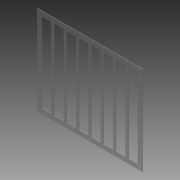
# Autodesk Inventor part: Back Plate Flat
Saved by Autodesk Inventor 2013 (Build 170138000, 138)
## iProperties
Created: 2013-02-02
Part Number: Back Plate Flat
Material: Polycarbonate, Clear
Document SubType Name: Modeling
Designer: Arpan
Mass: 34.1531 g
Surface Area: 558.316 cm^2
Volume: 38.2026 cm^3
Density: 0.894 g/cm^3
Author: Arpan
Autodesk Inventor part; units mm, degrees
ref_plane "YZ Plane" through (0, 0, 0) normal (1, 0, 0) x (0, 1, 0)
ref_plane "XZ Plane" through (0, 0, 0) normal (0, 1, 0) x (-1, 0, 0)
ref_plane "XY Plane" through (0, 0, 0) normal (0, 0, 1) x (1, 0, 0)
sketch "Sketch1" plane through (0, 0, 0) normal (0, 0, 1) x (1, 0, 0)
  line L0 (0, 0) -> (0, 238.1523)
  line L1 (0, 238.1523) -> (282.575, 238.1523)
  line L2 (282.575, 238.1523) -> (282.575, 0)
  line L3 (282.575, 0) -> (0, 0)
  line L4 (12.7, 225.4523) -> (38.1, 225.4523)
  line L5 (12.7, 225.4523) -> (12.7, 12.7)
  line L6 (12.7, 12.7) -> (38.1, 12.7)
  line L7 (38.1, 12.7) -> (38.1, 225.4523)
  line L8 (45.8107, 225.4523) -> (71.2107, 225.4523)
  line L9 (45.8107, 225.4523) -> (45.8107, 12.7)
  line L10 (45.8107, 12.7) -> (71.2107, 12.7)
  line L11 (71.2107, 12.7) -> (71.2107, 225.4523)
  line L12 (78.9214, 225.4523) -> (104.3214, 225.4523)
  line L13 (78.9214, 225.4523) -> (78.9214, 12.7)
  line L14 (78.9214, 12.7) -> (104.3214, 12.7)
  line L15 (104.3214, 12.7) -> (104.3214, 225.4523)
  line L16 (112.0321, 225.4523) -> (137.4321, 225.4523)
  line L17 (112.0321, 225.4523) -> (112.0321, 12.7)
  line L18 (112.0321, 12.7) -> (137.4321, 12.7)
  line L19 (137.4321, 12.7) -> (137.4321, 225.4523)
  line L20 (145.1429, 225.4523) -> (170.5429, 225.4523)
  line L21 (145.1429, 225.4523) -> (145.1429, 12.7)
  line L22 (145.1429, 12.7) -> (170.5429, 12.7)
  line L23 (170.5429, 12.7) -> (170.5429, 225.4523)
  line L24 (178.2536, 225.4523) -> (203.6536, 225.4523)
  line L25 (178.2536, 225.4523) -> (178.2536, 12.7)
  line L26 (178.2536, 12.7) -> (203.6536, 12.7)
  line L27 (203.6536, 12.7) -> (203.6536, 225.4523)
  line L28 (211.3643, 225.4523) -> (236.7643, 225.4523)
  line L29 (211.3643, 225.4523) -> (211.3643, 12.7)
  line L30 (211.3643, 12.7) -> (236.7643, 12.7)
  line L31 (236.7643, 12.7) -> (236.7643, 225.4523)
  line L32 (244.475, 225.4523) -> (269.875, 225.4523)
  line L33 (244.475, 225.4523) -> (244.475, 12.7)
  line L34 (244.475, 12.7) -> (269.875, 12.7)
  line L35 (269.875, 12.7) -> (269.875, 225.4523)
  dimension "d0" = 238.1523
  dimension "d1" = 282.575
  dimension "d2" = 25.4
  dimension "d3" = 12.7
  dimension "d5" = 12.7
  dimension "d6" = 12.7
  dimension "d9" = 33.1107
  constraints: 72 end point, 4 perpendicular, 3 parallel, 1 horizontal, 1 vertical, 56 other
  measures "d0" distance of L0.start L0.end
  measures "d1" distance of L0.end L1.end
  measures "d2" distance of L4.start L4.end
  measures "d3" distance between parallel lines of L1 L4
  measures "d5" distance between parallel lines of L3 L6
  measures "d6" distance between parallel lines of L0 L5
  measures "d9" distance of L4.start L8.start
extrude "Extrusion1" add sketch "Sketch1" along normal blind 1.5875
body "Solid1"
